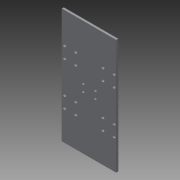
# Autodesk Inventor part: z-axis_mount_plate
Saved by Autodesk Inventor 2014 (Build 180170000, 170)
## iProperties
Created: 2014-08-18
Part Number: z-axis_mount_plate
Material: Generic
Document SubType Name: Modeling
Designer: Matthew
Density: 1 g/cm^3
Appearance: Default
Mass: 377.329 g
Surface Area: 1324.96 cm^2
Volume: 377.329 cm^3
Author: Matthew
Autodesk Inventor part; units mm, degrees
ref_plane "YZ Plane" through (0, 0, 0) normal (1, 0, 0) x (0, 1, 0)
ref_plane "XZ Plane" through (0, 0, 0) normal (0, 1, 0) x (-1, 0, 0)
ref_plane "XY Plane" through (0, 0, 0) normal (0, 0, 1) x (1, 0, 0)
sketch "Sketch1" plane through (0, 0, 0) normal (0, 1, 0) x (-1, 0, 0)
  line L0 (85, 179.925) -> (-85, 179.925)
  line L1 (-85, 179.925) -> (-85, -179.925)
  line L2 (-85, -179.925) -> (85, -179.925)
  line L3 (85, -179.925) -> (85, 179.925)
  line L4 (85, 179.925) -> (-85, -179.925) construction
  line L5 (-85, 179.925) -> (85, -179.925) construction
  point P0 (0, 0)
  dimension "d0" = 170
  dimension "d1" = 359.85
  constraints: 12 end point, 2 midpoint, 2 parallel, 1 horizontal, 1 perpendicular
  measures "d0" distance of L2.end L1.end
  measures "d1" distance of L0.end L1.end
extrude "Extrusion1" add sketch "Sketch1" along normal blind 6.35
sketch "Sketch2" plane through (0, 0, 0) normal (0, -1, 0) x (1, 0, 0)
  line L0 (-85, 179.925) -> (85, 179.925) projected
  line L1 (-85, -179.925) -> (-85, 179.925) projected
  line L2 (85, 179.925) -> (85, -179.925) projected
  line L3 (35, 43.4) -> (85, 43.4) construction
  line L4 (85, 43.4) -> (85, 91.4) construction
  line L5 (85, 91.4) -> (35, 91.4) construction
  line L6 (35, 91.4) -> (35, 43.4) construction
  line L7 (35, 43.4) -> (85, 91.4) construction
  line L8 (85, 43.4) -> (35, 91.4) construction
  line L9 (-85, 43.4) -> (-35, 43.4) construction
  line L10 (-35, 43.4) -> (-35, 91.4) construction
  line L11 (-35, 91.4) -> (-85, 91.4) construction
  line L12 (-85, 91.4) -> (-85, 43.4) construction
  line L13 (-85, 43.4) -> (-35, 91.4) construction
  line L14 (-35, 43.4) -> (-85, 91.4) construction
  line L15 (35, -91.4) -> (85, -91.4) construction
  line L16 (85, -91.4) -> (85, -43.4) construction
  line L17 (85, -43.4) -> (35, -43.4) construction
  line L18 (35, -43.4) -> (35, -91.4) construction
  line L19 (35, -91.4) -> (85, -43.4) construction
  line L20 (85, -91.4) -> (35, -43.4) construction
  line L21 (-85, -91.4) -> (-35, -91.4) construction
  line L22 (-35, -91.4) -> (-35, -43.4) construction
  line L23 (-35, -43.4) -> (-85, -43.4) construction
  line L24 (-85, -43.4) -> (-85, -91.4) construction
  line L25 (-85, -91.4) -> (-35, -43.4) construction
  line L26 (-35, -91.4) -> (-85, -43.4) construction
  line L27 (-24, -17.5) -> (24, -17.5) construction
  line L28 (24, -17.5) -> (24, 17.5) construction
  line L29 (24, 17.5) -> (-24, 17.5) construction
  line L30 (-24, 17.5) -> (-24, -17.5) construction
  line L31 (-24, -17.5) -> (24, 17.5) construction
  line L32 (24, -17.5) -> (-24, 17.5) construction
  point P0 (0, 0)
  point P1 (60, 67.4)
  point P2 (42.5, 84.9)
  point P3 (77.5, 84.9)
  point P4 (42.5, 49.9)
  point P5 (77.5, 49.9)
  point P6 (-60, 67.4)
  point P7 (-77.5, 84.9)
  point P8 (-42.5, 84.9)
  point P9 (-77.5, 49.9)
  point P10 (-42.5, 49.9)
  point P11 (60, -67.4)
  point P12 (42.5, -49.9)
  point P13 (77.5, -49.9)
  point P14 (42.5, -84.9)
  point P15 (77.5, -84.9)
  point P16 (-60, -67.4)
  point P17 (-77.5, -49.9)
  point P18 (-42.5, -49.9)
  point P19 (-77.5, -84.9)
  point P20 (-42.5, -84.9)
  point P21 (-19, 11)
  point P22 (19, 11)
  point P23 (-19, -11)
  point P24 (19, -11)
  dimension "d20" = 170
  dimension "d43" = 35
  dimension "d46" = 35
  dimension "d49" = 48
  dimension "d50" = 50
  dimension "d51" = 25
  dimension "d54" = 120
  dimension "d57" = 134.8
  dimension "d60" = 359.85
  dimension "d61" = 88.525
  dimension "d62" = 6.5
  dimension "d63" = 7.5
  dimension "d64" = 48
  dimension "d65" = 35
  dimension "d68" = 38
  dimension "d71" = 22
  dimension "d74" = 6.5
  dimension "d75" = 5
  dimension "d76" = 25.9
  constraints: 60 end point, 10 midpoint, 5 horizontal, 4 parallel, 3 vertical, 2 perpendicular, 51 other
  measures "d20" distance of L0.start L0.end
  measures "d43" distance of point (42.5, 84.9) point (77.5, 84.9)
  measures "d46" distance of point (42.5, 84.9) point (42.5, 49.9)
  measures "d49" distance of L5.end L3.start
  measures "d50" distance of L4.end L5.end
  measures "d51" distance from line of L2 point (60, 67.4)
  measures "d54" distance of L3.start L9.start
  measures "d57" distance of L3.start L15.start
  measures "d60" distance of L1.start L0.start
  measures "d61" distance between parallel lines of L0 L11
  measures "d62" distance from line of L5 point (42.5, 84.9)
  measures "d63" distance from line of L6 point (42.5, 84.9)
  measures "d64" distance of L28.end L29.end
  measures "d65" distance of L27.end L28.end
  measures "d68" distance of point (-19, 11) point (19, 11)
  measures "d71" distance of point (-19, 11) point (-19, -11)
  measures "d74" distance from line of L29 point (-19, 11)
  measures "d75" distance from line of L28 point (19, 11)
  measures "d76" distance between parallel lines of L3 L29
hole "Hole2" at (-19, 0, 11) at (19, 0, 11) at (19, 0, -11) at (-19, 0, -11) direction (0, 1, 0) diameter 4 depth 8 tip angle 118
hole "Hole3" at (42.5, 0, 84.9) at (77.5, 0, 84.9) at (42.5, 0, 49.9) at (77.5, 0, 49.9) at (-42.5, 0, 49.9) at (-77.5, 0, 49.9) at (-42.5, 0, 84.9) at (-77.5, 0, 84.9) at (77.5, 0, -84.9) at (42.5, 0, -84.9) at (77.5, 0, -49.9) at (42.5, 0, -49.9) at (-42.5, 0, -84.9) at (-77.5, 0, -84.9) at (-42.5, 0, -49.9) at (-77.5, 0, -49.9) direction (0, 1, 0) diameter 5 depth 8 tip angle 118
hole "Hole4" at (-19, 0, 11) at (19, 0, 11) at (19, 0, -11) at (-19, 0, -11) direction (0, 1, 0) diameter 9.75 depth 5
hole "Hole5" at (-77.5, 0, 49.9) at (-42.5, 0, 49.9) at (-42.5, 0, 84.9) at (-77.5, 0, 84.9) at (42.5, 0, 84.9) at (77.5, 0, 84.9) at (77.5, 0, 49.9) at (42.5, 0, 49.9) at (77.5, 0, -49.9) at (42.5, 0, -49.9) at (42.5, 0, -84.9) at (77.5, 0, -84.9) at (-42.5, 0, -84.9) at (-42.5, 0, -49.9) at (-77.5, 0, -49.9) at (-77.5, 0, -84.9) direction (0, 1, 0) diameter 11.2 depth 6
equation "\"d51\" = 0.5 * d50"
equation "\"d61\" = -0.5 * d49 + 0.5 * d60 - 0.5 * d57"
equation "\"d74\" = -0.5 * d71 + 0.5 * d65"
equation "\"d75\" = -0.5 * d68 + 0.5 * d64"
body "Solid1"
